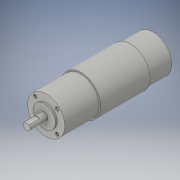
# Autodesk Inventor part: motor
Saved by Autodesk Inventor 2016 (Build 200138000, 138)
## iProperties
Created: 2015-09-28
Part Number: motor
Material: Generic
Document SubType Name: Modeling
Designer: Mack
Density: 1 g/cm^3
Appearance: Default
Author: Mack
Autodesk Inventor part; units mm, degrees
ref_plane "YZ Plane" through (0, 0, 0) normal (1, 0, 0) x (0, 1, 0)
ref_plane "XZ Plane" through (0, 0, 0) normal (0, 1, 0) x (-1, 0, 0)
ref_plane "XY Plane" through (0, 0, 0) normal (0, 0, 1) x (1, 0, 0)
sketch "Sketch1" plane through (0, 0, 0) normal (0, 0, 1) x (1, 0, 0)
  circle A0 centre (0, 0) radius 22.5
  dimension "d0" = 45
  constraints: 1 centre point, 1 coincident
  measures "d0" diameter of A0
extrude "Extrusion1" add sketch "Sketch1" along normal blind 66
sketch "Sketch2" plane through (0, 0, 66) normal (0, 0, 1) x (1, 0, 0)
  circle A0 centre (0, 0) radius 21
  dimension "d3" = 42
  constraints: 1 centre point, 1 coincident
  measures "d3" diameter of A0
extrude "Extrusion2" add sketch "Sketch2" along normal blind 39.2
sketch "Sketch3" plane through (0, 0, 105.2) normal (0, 0, 1) x (1, 0, 0)
  circle A0 centre (0, 0) radius 12.5
  dimension "d6" = 25
  constraints: 1 centre point, 1 coincident
  measures "d6" diameter of A0
extrude "Extrusion3" add sketch "Sketch3" along normal blind 2
sketch "Sketch4" plane through (0, 0, 107.2) normal (0, 0, 1) x (1, 0, 0)
  circle A0 centre (0, 0) radius 4
  dimension "d9" = 8
  constraints: 1 centre point, 1 coincident
  measures "d9" diameter of A0
extrude "Extrusion4" add sketch "Sketch4" along normal blind 20
sketch "Sketch5" plane through (0, 0, 127.2) normal (0, 0, 1) x (1, 0, 0)
  line L0 (-2.6886, 3) -> (2.6458, 3)
  circle A0 centre (0, 0) radius 4 projected
  arc A1 (2.6458, 3) -> (-2.6458, 3) centre (0, 0) ccw
  dimension "d12" = 3
  constraints: 2 end point, 2 point on circle, 1 centre point, 1 coincident, 1 horizontal, 1 point on line, 2 other
  measures "d12" distance from line of point (0, 0) L0
extrude "Extrusion5" cut sketch "Sketch5" against normal blind 12 contours A0 L0 picked at (0.5822, 3.4764)
sketch "Sketch6" plane through (0, 0, 105.2) normal (0, 0, 1) x (1, 0, 0)
  point P0 (0, 0)
  point P1 (-12.3747, 12.374)
  point P2 (-12.374, -12.3747)
  point P3 (12.3747, -12.374)
  point P4 (12.374, 12.3747)
  dimension "d15" = 17.5
  dimension "d16" = 12.374
  dimension "d19" = 360
  constraints: 5 other
  measures "d15" distance of point (0, 0) point (-12.375, 12.374)
  measures "d16" vertical distance of point (0, 0) point (-12.375, 12.374)
hole "Hole1" at (-12.3747, 12.374, 105.2) at (-12.374, -12.3747, 105.2) at (12.3747, -12.374, 105.2) at (12.374, 12.3747, 105.2) direction (0, 0, -1) diameter 3.25 depth 7 tip angle 118 counterbore diameter 4 counterbore depth 1
sketch "Sketch7" plane through (0, 0, 0) normal (0, 0, -1) x (-1, 0, 0)
  circle A0 centre (0, 0) radius 21 projected
  circle A1 centre (0, 0) radius 13.921
  circle A2 centre (0, 0) radius 4 projected
  circle A3 centre (0, 0) radius 21
  circle A4 centre (0, 0) radius 22.5
  dimension "d28" = 42
  constraints: 3 centre point, 3 coincident
  measures "d28" diameter of A3
extrude "Extrusion6" cut sketch "Sketch7" against normal blind 10 contours A4
sketch "Sketch8" plane through (0, 0, 0) normal (0, 0, -1) x (-1, 0, 0)
  circle A0 centre (0, 0) radius 21
  constraints: 1 centre point, 1 coincident
extrude "Extrusion7" add sketch "Sketch8" along normal blind 16.1
body "Solid1"
